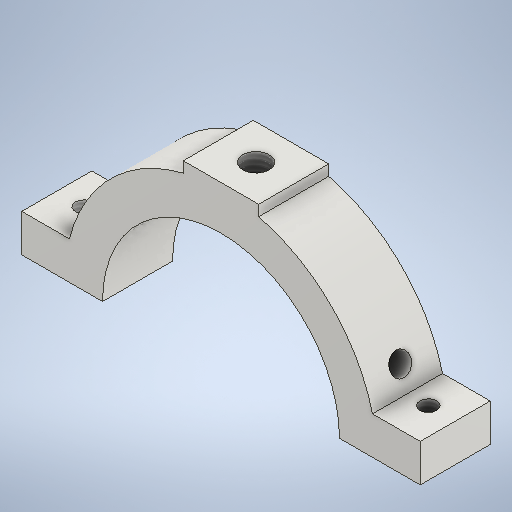
# Autodesk Inventor part: 29 - Sheave Strap 1
Saved by Autodesk Inventor 2025.2 (Build 292293000, 293)
## iProperties
Created: 2025-07-30
Part Number: 29 - Sheave Strap 1
Material: Steel AISI 1020 107 HR
Document SubType Name: Modeling
Designer: bless
Density: 7.87 g/cm^3
Appearance: Steel
Author: bless
Autodesk Inventor part; units mm, degrees
ref_plane "YZ Plane" through (0, 0, 0) normal (1, 0, 0) x (0, 1, 0)
ref_plane "XZ Plane" through (0, 0, 0) normal (0, 1, 0) x (-1, 0, 0)
sketch "Sketch1" plane through (0, 0, 0) normal (0, 0, 1) x (1, 0, 0)
  arc A0 (11, 0) -> (-11, 0) centre (0, 0) ccw
  arc A1 (14.0712, 3.5) -> (-14.0712, 3.5) centre (0, 0) ccw
  line L0 (-11, 0) -> (-18.5, 0)
  line L1 (-18.5, 0) -> (-18.5, 3.5)
  line L2 (11, 0) -> (18.5, 0)
  line L3 (18.5, 0) -> (18.5, 3.5)
  line L4 (-18.5, 3.5) -> (-14.0712, 3.5)
  line L5 (18.5, 3.5) -> (14.0712, 3.5)
  line L6 (-3.5, 15.0712) -> (3.5, 15.0712)
  line L7 (3.5, 15.0712) -> (3.5, 14.0712)
  line L8 (-3.5, 15.0712) -> (-3.5, 14.0712)
  point P0 (0, 15.0712)
  dimension "d2" = 11
  dimension "d3" = 14.5
  dimension "d4" = 7.5
  dimension "d5" = 3.5
  dimension "d6" = 18.5
  dimension "d7" = 7
  dimension "d8" = 1
  constraints: 18 end point, 6 point on circle, 4 horizontal, 3 equal length, 2 centre point, 2 coincident, 2 perpendicular, 1 midpoint, 1 parallel, 1 point on line, 1 vertical, 1 vertical alignment
  measures "d2" radius of A0
  measures "d3" radius of A1
  measures "d4" distance of L0.start L0.end
  measures "d5" distance of L2.end L3.end
  measures "d6" distance from line of L1 point (0, 0)
  measures "d7" distance of L6.start L6.end
  measures "d8" distance of L6.end L7.end
extrude "Extrusion1" add sketch "Sketch1" along normal blind 6.5
sketch "Sketch2" plane through (0, 0, 6.5) normal (0, 0, 1) x (1, 0, 0)
  line L0 (-18.5, 3.5) -> (-18.5, 0) projected
  line L1 (-18.5, 0) -> (-11, 0) projected
  arc A0 (11, 0) -> (-11, 0) centre (0, 0) ccw projected
  line L2 (11, 0) -> (18.5, 0) projected
  line L3 (18.5, 0) -> (18.5, 3.5) projected
  line L4 (18.5, 3.5) -> (14.0712, 3.5) projected
  arc A1 (14.0712, 3.5) -> (3.5, 14.0712) centre (0, 0) ccw projected
  line L5 (3.5, 14.0712) -> (3.5, 15.0712) projected
  line L6 (3.5, 15.0712) -> (-3.5, 15.0712) projected
  line L7 (-3.5, 15.0712) -> (-3.5, 14.0712) projected
  arc A2 (-3.5, 14.0712) -> (-14.0712, 3.5) centre (0, 0) ccw projected
  line L8 (-14.0712, 3.5) -> (-18.5, 3.5) projected
  line L9 (0, 0) -> (18.5, 0)
  line L10 (0, 0) -> (23.4857, 9.7281)
  dimension "d11" = 22.5
  constraints: 4 end point, 1 horizontal
  measures "d11" angle of L9 L10
ref_plane "Work Plane2" through (11.866, 9.4714, 3.25) normal (0.9239, 0.3827, 0) x (-0.3827, 0.9239, 0)
ref_plane "Work Plane1" through (-11, 0, 3.25) normal (0.9239, 0.3827, 0) x (-0.3827, 0.9239, 0)
sketch "Sketch3" plane through (11.866, 9.4714, 3.25) normal (0.9239, 0.3827, 0) x (-0.3827, 0.9239, 0)
  line L0 (-4.2095, 3.25) -> (-11.2892, 3.25) projected
  line L1 (-6.3608, -3.25) -> (7.4512, -3.25) projected
  line L2 (7.4512, -3.25) -> (7.4512, 3.25) projected
  line L3 (-6.3608, 3.25) -> (7.4512, 3.25) projected
  line L4 (-6.3608, -3.25) -> (-6.3608, 3.25) projected
  line L5 (-11.2892, -3.25) -> (-8.0556, -3.25) projected
  line L6 (-8.0556, -3.25) -> (-8.0556, 3.25) projected
  line L7 (-11.2892, 3.25) -> (-8.0556, 3.25) projected
  line L8 (-11.2892, -3.25) -> (-11.2892, 3.25) projected
  line L9 (-8.0556, -3.25) -> (-6.3608, -3.25) projected
  line L10 (-6.3608, -3.25) -> (-6.3608, 3.25) projected
  line L11 (-8.0556, 3.25) -> (-6.3608, 3.25) projected
  line L12 (-8.0556, -3.25) -> (-8.0556, 3.25) projected
  point P0 (-4.2095, -3.25)
  point P1 (-4.2095, 0)
  point P2 (-4.2095, 3.25)
  dimension "d13" = 3.25
  dimension "d14" = 11.6608
  measures "d13" distance from line of L1 point (-4.21, 0)
  measures "d14" distance from line of point (-4.21, 0) L2
hole "Hole1" at (13.4769, 5.5823, 3.25) direction (-0.9239, -0.3827, 0) diameter 2 end through all
sketch "Sketch4" plane through (-3.5, 15.0712, 0) normal (0, 1, 0) x (1, 0, 0)
  line L0 (7, 0) -> (0, 0) projected
  line L1 (-15, 0) -> (-15, -6.5) projected
  point P0 (3.5, 0)
  point P1 (3.5, -3.25)
  point P2 (-15, -3.25)
  dimension "d22" = 18.5
  dimension "d23" = 3.25
  constraints: 1 midpoint
  measures "d22" distance of point (-15, -3.25) point (3.5, -3.25)
  measures "d23" distance from line of point (3.5, -3.25) L0
hole "Hole2" at (0, 15.0712, 3.25) direction (0, -1, 0) diameter 2.459 end through all thread size "M3x0.5" class "6H" standard "ANSI Metric M Profile"
sketch "Sketch5" plane through (-18.5, 3.5, 0) normal (0, 1, 0) x (1, 0, 0)
  line L0 (4.4288, 0) -> (0, 0) projected
  line L1 (0, 0) -> (0, -6.5) projected
  line L2 (37, 0) -> (37, -6.5) projected
  line L3 (37, 0) -> (32.5712, 0) projected
  point P0 (18.5, 0)
  point P1 (2.5, -3.25)
  point P2 (34.5, -3.25)
  point P3 (0, -3.25)
  dimension "d31" = 2.5
  dimension "d32" = 2.5
  dimension "d33" = 3.25
  dimension "d34" = 3.25
  constraints: 1 midpoint
  measures "d31" distance from line of L2 point (34.5, -3.25)
  measures "d32" distance of point (0, -3.25) point (2.5, -3.25)
  measures "d33" distance from line of point (34.5, -3.25) L3
  measures "d34" distance from line of L0 point (2.5, -3.25)
hole "Hole3" at (-16, 3.5, 3.25) at (16, 3.5, 3.25) direction (0, -1, 0) diameter 1.567 end through all thread size "M2x0.4" class "6H" standard "ANSI Metric M Profile"
body "Solid1"
